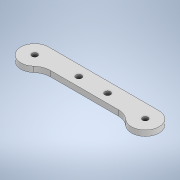
# Autodesk Inventor part: prig to kauri conversion plate
Saved by Autodesk Inventor 2020 (Build 240168000, 168)
## iProperties
Created: 2022-05-24
Part Number: prig to kauri conversion plate
Material: Generic
Document SubType Name: Modeling
Designer: Steven
Density: 1 g/cm^3
Appearance: Default
Author: Steven
Autodesk Inventor part; units mm, degrees
ref_plane "YZ Plane" through (0, 0, 0) normal (1, 0, 0) x (0, 1, 0)
ref_plane "XZ Plane" through (0, 0, 0) normal (0, 1, 0) x (-1, 0, 0)
ref_plane "XY Plane" through (0, 0, 0) normal (0, 0, 1) x (1, 0, 0)
sketch "Sketch1" plane through (0, 0, 0) normal (0, 1, 0) x (-1, 0, 0)
  circle A0 centre (-16.9706, -0.5878) radius 1.5
  circle A1 centre (16.9706, -0.5878) radius 1.5
  circle A2 centre (30, -5.1319) radius 1.5
  circle A3 centre (-30, -5.1319) radius 1.5
  circle A4 centre (16.9706, -0.5878) radius 5 construction
  circle A5 centre (-16.9706, -0.5878) radius 5 construction
  arc A6 (-31.1155, 2.2846) -> (-30, -12.6319) centre (-30, -5.1319) ccw
  arc A7 (30, -12.6319) -> (31.1155, 2.2846) centre (30, -5.1319) ccw
  line L0 (30, -12.6319) -> (-30, -12.6319)
  line L1 (-16.9706, 4.4122) -> (16.9706, 4.4122)
  line L2 (-16.9706, 4.4122) -> (-31.1155, 2.2846)
  line L3 (16.9706, 4.4122) -> (31.1155, 2.2846)
  arc A8 (31.1155, 2.2846) -> (23.1456, -2.0878) centre (30, -5.1319) ccw
  arc A9 (-30, -12.6319) -> (-23.1456, -2.0878) centre (-30, -5.1319) ccw construction
  line L4 (0, 4.2106) -> (0, -4.2106) construction
  line L5 (0, -4.2106) -> (3.1574, -4.2106) construction
  line L6 (0, -4.2106) -> (0, -12.6319) construction
  circle A10 centre (0, 0) radius 1.55
  line L7 (0, -8.4213) -> (15.6117, -8.4213) construction
  line L8 (0, -8.4213) -> (-15.6117, -8.4213) construction
  circle A11 centre (7.8058, -8.4213) radius 1.55 construction
  circle A12 centre (-7.8058, -8.4213) radius 1.55 construction
  line L9 (16.9706, -2.0878) -> (-16.9706, -2.0878)
  line L10 (16.9706, -2.0878) -> (23.1456, -2.0878)
  line L11 (-16.9706, -2.0878) -> (-23.1456, -2.0878)
  arc A13 (-23.1456, -2.0878) -> (-31.1155, 2.2846) centre (-30, -5.1319) ccw
  arc A14 (23.1456, -2.0878) -> (30, -12.6319) centre (30, -5.1319) ccw construction
  line L12 (7.8058, -12.6319) -> (7.8058, -2.0878) construction
  line L13 (-7.8058, -12.6319) -> (-7.8058, -2.0878) construction
  line L14 (7.8058, -6.8713) -> (-7.8058, -6.8713) construction
  circle A15 centre (-7.8058, -6.8713) radius 1.55
  circle A16 centre (7.8058, -6.8713) radius 1.55
  point P0 (0, 0)
  dimension "d0" = 10
  dimension "d1" = 10
  dimension "d5" = 3.1
  dimension "d6" = 3.1
  dimension "d2" = 15
  dimension "d3" = 15
  dimension "d4" = 3.1
  dimension "d10" = 3.1
  dimension "d11" = 3.1
  constraints: 30 end point, 12 point on circle, 11 centre point, 9 point on line, 6 coincident, 6 vertical alignment, 5 horizontal, 5 midpoint, 3 tangent, 2 perpendicular, 12 other
  measures "d2" diameter of A6
  measures "d3" diameter of A7
  measures "d4" diameter of A10
  measures "d10" diameter of A15
  measures "d11" diameter of A16
extrude "Extrusion1" add sketch "Sketch1" along normal blind 3 contours L9 L10 A8 A7 L0 A6 A13 L11
fillet "Fillet1" radius 10 2 edges at (-23.1456, 1.5, -2.0878) (23.1456, 1.5, -2.0878)
body "Solid1"
